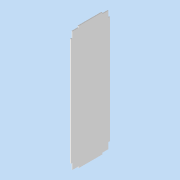
# Autodesk Inventor part: Acrly_Wand_1
Saved by Autodesk Inventor 2022 (Build 260153000, 153)
## iProperties
Created: 2021-12-15
Part Number: Acrly_Wand_1
Material: Generic
Document SubType Name: Modeling
Designer: Fabijansven
Density: 1 g/cm^3
Appearance: Default
Author: Fabijansven
Autodesk Inventor part; units mm, degrees
ref_plane "YZ Plane" through (0, 0, 0) normal (1, 0, 0) x (0, 1, 0)
ref_plane "XZ Plane" through (0, 0, 0) normal (0, 1, 0) x (-1, 0, 0)
ref_plane "XY Plane" through (0, 0, 0) normal (0, 0, 1) x (1, 0, 0)
sketch "Sketch1" plane through (0, 0, 0) normal (1, 0, 0) x (0, 1, 0)
  line L0 (0, 0) -> (642, 0)
  line L1 (642, 0) -> (642, -204)
  line L2 (642, -204) -> (0, -204)
  line L3 (0, -204) -> (0, 0)
  line L4 (642, 0) -> (634, 0)
  line L5 (634, 0) -> (634, -40)
  line L6 (634, -40) -> (642, -40)
  line L7 (642, -40) -> (642, 0)
  line L8 (642, 0) -> (602, 0)
  line L9 (602, 0) -> (602, -8)
  line L10 (602, -8) -> (642, -8)
  line L11 (642, -8) -> (642, 0)
  line L12 (856.5319, -102) -> (-65.1606, -102) construction
  line L13 (321, 165.682) -> (321, -1074.2454) construction
  line L14 (642, -204) -> (634, -204)
  line L15 (634, -204) -> (634, -164)
  line L16 (634, -164) -> (642, -164)
  line L17 (642, -164) -> (642, -204)
  line L18 (642, -204) -> (602, -204)
  line L19 (602, -204) -> (602, -196)
  line L20 (602, -196) -> (642, -196)
  line L21 (642, -196) -> (642, -204)
  line L22 (0, 0) -> (0, -204)
  line L23 (0, 0) -> (8, 0)
  line L24 (8, 0) -> (8, -40)
  line L25 (8, -40) -> (0, -40)
  line L26 (0, -40) -> (0, 0)
  line L27 (0, 0) -> (40, 0)
  line L28 (40, 0) -> (40, -8)
  line L29 (40, -8) -> (0, -8)
  line L30 (0, -8) -> (0, 0)
  line L31 (8, -164) -> (0, -164)
  line L32 (40, -196) -> (0, -196)
  line L33 (0, -204) -> (8, -204)
  line L34 (8, -204) -> (8, -164)
  line L35 (0, -164) -> (0, -204)
  line L36 (0, -204) -> (40, -204)
  line L37 (40, -204) -> (40, -196)
  line L38 (0, -196) -> (0, -204)
  point P0 (40, -204)
  point P1 (602, -204)
  point P2 (634, -196)
  point P3 (642, -164)
  point P4 (642, -40)
  point P5 (634, -8)
  point P6 (602, 0)
  point P7 (40, 0)
  point P8 (8, -8)
  point P9 (0, -40)
  point P10 (0, -164)
  point P11 (8, -196)
  dimension "d0" = 642
  dimension "d1" = 204
  dimension "d2" = 40
  dimension "d3" = 40
  dimension "d4" = 8
  dimension "d5" = 8
  dimension "d6" = 102
  dimension "d7" = 321
  constraints: 78 end point, 18 symmetric about line, 6 parallel, 4 horizontal, 3 perpendicular, 1 vertical
  measures "d0" distance of L1.end L2.end
  measures "d1" distance of L0.end L1.end
  measures "d2" distance of L4.end L5.end
  measures "d3" distance of L9.end L10.end
  measures "d4" distance of L8.end L9.end
  measures "d5" distance of L5.end L6.end
  measures "d6" distance between parallel lines of L0 L12
  measures "d7" distance between parallel lines of L3 L13
extrude "Extrusion1" add sketch "Sketch1" along normal blind 5 contours L0 L9 L10 L5 L6 L1 L16 L15 L20 L19 L2 L37 L32 L34 L31 L3 L25 L24 L29 L28
equation "\"d6\" = 0.5 * d1"
equation "\"d7\" = 0.5 * d0"
body "Solid1"
